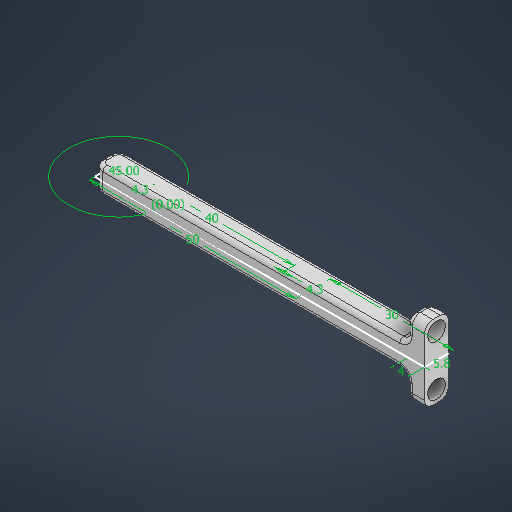
# Autodesk Inventor part: Arm
Saved by Autodesk Inventor 2026.2 (Build 302298000, 298)
## iProperties
Created: 2026-01-26
Part Number: Arm
Material: Generic
Document SubType Name: Modeling
Designer: Cobble
Density: 1 g/cm^3
Appearance: Default
Author: Cobble
Autodesk Inventor part; units mm, degrees
ref_plane "YZ Plane" through (0, 0, 0) normal (1, 0, 0) x (0, 1, 0)
ref_plane "XZ Plane" through (0, 0, 0) normal (0, 1, 0) x (-1, 0, 0)
ref_plane "XY Plane" through (0, 0, 0) normal (0, 0, 1) x (1, 0, 0)
sketch "Sketch1" plane through (0, 0, 0) normal (0, 0, 1) x (1, 0, 0)
  line L0 (0, 0) -> (30, 0)
  line L1 (30, 0) -> (30, 5.8)
  line L2 (30, 5.8) -> (0, 5.8)
  line L3 (0, 5.8) -> (0, 0)
  line L4 (0, 5.8) -> (-50, 5.8)
  line L5 (-50, 5.8) -> (-50, 0)
  line L6 (-50, 0) -> (0, 0)
  line L7 (0, 0) -> (0, 5.8)
  line L8 (30, 5.8) -> (26, 5.8)
  line L9 (26, 5.8) -> (26, 0)
  line L10 (26, 0) -> (30, 0)
  line L11 (30, 0) -> (30, 5.8)
  line L12 (-50, 5.8) -> (-44.2, 0)
  line L13 (-50, 5.8) -> (-41.7976, 5.8) construction
  circle A0 centre (-47.1, 2.9) radius 2.15
  line L14 (-47.1, 2.9) -> (-7.1, 2.9)
  line L15 (-47.1, 2.9) -> (-7.1, 2.9) construction
  circle A1 centre (-7.1, 2.9) radius 2.15
  dimension "d0" = 30
  dimension "d1" = 5.8
  dimension "d2" = 50
  dimension "d3" = 4
  dimension "d4" = 45
  dimension "d5" = 4.3
  dimension "d6" = 40
  dimension "d7" = 0
  dimension "d8" = 4.3
  constraints: 32 end point, 7 parallel, 5 horizontal, 3 perpendicular, 3 point on line, 2 centre point, 2 equal length, 1 coincident, 1 midpoint
  measures "d0" distance of L2.end L1.end
  measures "d1" distance of L1.end L0.end
  measures "d2" distance of L6.end L5.end
  measures "d3" distance of L10.end L9.end
  measures "d4" angle of L12 L13
  measures "d5" diameter of A0
  measures "d6" distance of L14.start L14.end
  measures "d7" distance between parallel lines of L14 L15
  measures "d8" diameter of A1
extrude "Extrusion1" add sketch "Sketch1" along normal mid plane 6 contours L3 L2 L9 L0 | L6 L12 A0 L4 L3 | L9 L2 L1 L0 | L6 L5 L12 A0 | A0 L12 | L12 L14 A0 | A0 L14 L12 | A1
extrude "Extrusion2" add sketch "Sketch1" along normal mid plane 18 contours L9 L2 L1 L0
sketch "Sketch2" plane through (30, 0, 9) normal (1, 0, 0) x (0, 0, -1)
  line L0 (18, 5.8) -> (0, 5.8) projected
  line L1 (0, 0) -> (0, 5.8) projected
  line L2 (18, 0) -> (0, 0) projected
  line L3 (18, 5.8) -> (18, 0) projected
  line L4 (0, 5.8) -> (5.8, 0)
  line L5 (18, 0) -> (0, 0) projected
  line L6 (0, 5.8) -> (8.2024, 5.8) construction
  line L7 (18, 5.8) -> (12.2, 0)
  line L8 (18, 5.8) -> (26.2024, 5.8) construction
  circle A0 centre (2.9, 2.9) radius 2.15
  circle A1 centre (15.1, 2.9) radius 2.15
  point P0 (9, 0)
  dimension "d13" = 45
  dimension "d14" = 135
  dimension "d15" = 4.3
  dimension "d16" = 4.3
  constraints: 8 end point, 2 centre point, 2 equal length, 2 horizontal, 2 midpoint, 2 point on line
  measures "d13" angle of L4 L6
  measures "d14" angle of L7 L8
  measures "d15" diameter of A0
  measures "d16" diameter of A1
extrude "Extrusion3" cut sketch "Sketch2" against normal blind 18 contours A1 L7 | L7 A1 | A0 L4 | L4 A0
fillet "Fillet1" radius 2 4 edges at (28, 5.8, 9) (28, 0, 9) (28, 5.8, -9) (28, 0, -9)
fillet "Fillet2" radius 2 2 edges at (-50, 5.8, 0) (-50, 0, 0)
fillet "Fillet3" radius 2 2 edges at (26, 2.9, 3) (26, 2.9, -3)
fillet "Fillet4" radius 1 24 edges at (-12, 5.8, 3) (25.4142, 5.8, 3.5858) (26, 5.8, 6) (26, 5.2142, 8.4142) (26, 2.9, 9) (26, 0.5858, 8.4142) (26, 0, 6) (25.4142, 0, 3.5858) (-12, 0, 3) (-49.4142, 0.5858, 3) (-50, 2.9, 3) (-49.4142, 5.2142, 3) (25.4142, 5.8, -3.5858) (26, 5.8, -6) (26, 5.2142, -8.4142) (26, 2.9, -9) (26, 0.5858, -8.4142) (26, 0, -6) (25.4142, 0, -3.5858) (-12, 0, -3) (-49.4142, 0.5858, -3) (-50, 2.9, -3) (-49.4142, 5.2142, -3) (-12, 5.8, -3)
body "Solid1"
